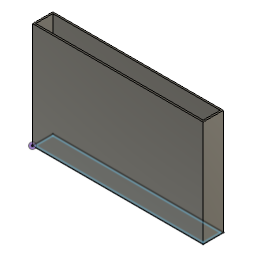
Auffangbehaelter (Autodesk Fusion 360 design; units mm, degrees)
part number: 2025-12-02-23-05-34-915
Autodesk Fusion 360 part; units mm, degrees
sketch "Skizze1" plane through (0, 0, 0) normal (0, 0, 1) x (1, 0, 0)
  line L0 (0, 0) -> (200, 0)
  line L1 (200, 0) -> (200, 24)
  line L2 (200, 24) -> (0, 24)
  line L3 (0, 24) -> (0, 0)
  line L4 (2, 2) -> (198, 2)
  line L5 (198, 2) -> (198, 22)
  line L6 (198, 22) -> (2, 22)
  line L7 (2, 22) -> (2, 2)
  dimension "d1" = 200
  dimension "d2" = 24
  constraint horizontal L0
  constraint vertical L1
  constraint horizontal L2
  constraint vertical L3
  constraint coincident L0.start L3.end
  constraint horizontal L4
  constraint vertical L5
  constraint horizontal L6
  constraint vertical L7
  measures "d1" distance of L0.start L0.end
  measures "d2" distance of L0.start L2.end
extrude "Extrusion1" add sketch "Skizze1" along normal blind 2 contours L4 L5 L6 L7
extrude "Extrusion2" add sketch "Skizze1" along normal blind 124
